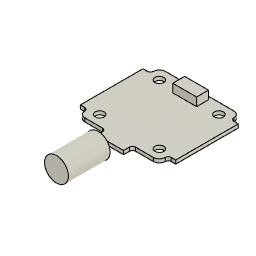
15A ESC v4 (Autodesk Fusion 360 design; units mm, degrees)
Autodesk Fusion 360 part; units mm, degrees
note: some values were not read from the file. Set by a fixed rule: which sketch regions a step uses.
sketch "Sketch1" plane through (0, 0, 0) normal (0, 0, 1) x (1, 0, 0)
  line L0 (-10, 10) -> (10, 10) construction
  line L1 (10, 10) -> (10, -10) construction
  line L2 (10, -10) -> (-10, -10) construction
  line L3 (-10, -10) -> (-10, 10) construction
  line L4 (-10, 10) -> (10, -10) construction
  line L5 (10, 10) -> (-10, -10) construction
  circle A0 centre (-10, 10) radius 1.5
  circle A1 centre (10, 10) radius 1.5
  circle A2 centre (10, -10) radius 1.5
  circle A3 centre (-10, -10) radius 1.5
  line L6 (-13.5, 13.5) -> (13.5, 13.5)
  line L7 (13.5, 13.5) -> (13.5, -13.5)
  line L8 (13.5, -13.5) -> (-13.5, -13.5)
  line L9 (-13.5, -13.5) -> (-13.5, 13.5)
  line L10 (-13.5, 13.5) -> (13.5, -13.5) construction
  line L11 (13.5, 13.5) -> (-13.5, -13.5) construction
  line L12 (-4.5, -16.5) -> (4.5, -16.5)
  line L13 (4.5, -16.5) -> (4.5, -13.5)
  line L14 (4.5, -13.5) -> (-4.5, -13.5)
  line L15 (-4.5, -13.5) -> (-4.5, -16.5)
  line L16 (-16, 10.5) -> (-13.5, 10.5)
  line L17 (-13.5, 10.5) -> (-13.5, -10.5)
  line L18 (-13.5, -10.5) -> (-16, -10.5)
  line L19 (-16, -10.5) -> (-16, 10.5)
  line L20 (0, 2.5) -> (0, 20)
  line L21 (13.5, 10.5) -> (13.5, -10.5)
  line L22 (13.5, -10.5) -> (16, -10.5)
  line L23 (16, -10.5) -> (16, 10.5)
  line L24 (16, 10.5) -> (13.5, 10.5)
  line L25 (-4, 12.5) -> (4, 12.5)
  line L26 (4, 12.5) -> (4, 8.5)
  line L27 (4, 8.5) -> (-4, 8.5)
  line L28 (-4, 8.5) -> (-4, 12.5)
  line L29 (-4, 12.5) -> (4, 8.5) construction
  line L30 (4, 12.5) -> (-4, 8.5) construction
  point P0 (0, 10.5)
  dimension "d1" = 20
  dimension "d2" = 20
  dimension "d3" = 3
  dimension "d4" = 27
  dimension "d5" = 27
  dimension "d6" = 9
  dimension "d7" = 3
  dimension "d8" = 2.5
  dimension "d9" = 21
  dimension "d12" = 8
  dimension "d13" = 4
  dimension "d14" = 1
  constraint horizontal L0
  constraint perpendicular L0 L1
  constraint parallel L0 L2
  constraint parallel L1 L3
  constraint coincident L4 origin
  constraint coincident L5 origin
  constraint coincident L0.start L3.end
  constraint coincident L0.end L1.start
  constraint coincident L1.end L2.start
  constraint coincident L2.end L3.start
  constraint equal A1 A3
  constraint equal A1 A2
  constraint equal A0 A2
  constraint horizontal L6
  constraint perpendicular L6 L7
  constraint parallel L6 L8
  constraint parallel L7 L9
  constraint coincident L10 origin
  constraint coincident L11 origin
  constraint horizontal L12
  constraint vertical L13
  constraint horizontal L14
  constraint vertical L15
  constraint midpoint L8 L14
  constraint horizontal L16
  constraint vertical L17
  constraint horizontal L18
  constraint vertical L19
  constraint midpoint L9 L17
  constraint symmetric L16.start L20 L23.end
  constraint symmetric L16.end L20 L21.start
  constraint symmetric L17.end L20 L21.end
  constraint symmetric L18.end L20 L22.end
  constraint horizontal L25
  constraint perpendicular L25 L26
  constraint parallel L25 L27
  constraint parallel L26 L28
  constraint coincident L29 P0
  constraint coincident L30 P0
  constraint coincident L20 P0
  measures "d1" distance of L1.end L2.end
  measures "d2" distance of L0.end L1.end
  measures "d3" diameter of A0
  measures "d4" distance of L7.end L8.end
  measures "d5" distance of L6.end L7.end
  measures "d6" distance of L12.start L12.end
  measures "d7" distance of L12.start L14.end
  measures "d8" distance of L16.start L16.end
  measures "d9" distance of L16.start L18.end
  measures "d12" distance of L26.end L27.end
  measures "d13" distance of L25.end L26.end
  measures "d14" distance of L6 L25
extrude "Extrude1" add sketch "Sketch1" along normal blind 1.2 makes body 1
extrude "Extrude2" add sketch "Sketch1" along normal blind 4 contours L20 L25 L27 L28 | L20 L25 L26 L27 bodies 1
fillet "Fillet1" radius 1 6 edges at (4.5, -13.5, 0.6) (-4.5, -13.5, 0.6) (-13.5, -10.5, 0.6) (-13.5, 10.5, 0.6) (13.5, 10.5, 0.6) (13.5, -10.5, 0.6) on bodies 1
fillet "Fillet2" radius 2 4 edges at (-13.5, -13.5, 0.6) (13.5, -13.5, 0.6) (13.5, 13.5, 0.6) (-13.5, 13.5, 0.6) on bodies 1
sketch "Sketch2" plane through (0, -16.5, 0) normal (0, -1, 0) x (1, 0, 0)
  line L0 (-4.5, 0) -> (4.5, 0)
  line L1 (4.5, 0) -> (4.5, 1.2)
  line L2 (4.5, 1.2) -> (-4.5, 1.2)
  line L3 (-4.5, 1.2) -> (-4.5, 0)
  circle A0 centre (0, 2.5) radius 4
  line L4 (0, 2.5) -> (0, 0) construction
  dimension "d23" = 8
  dimension "d24" = 2.5
  constraint coincident A0.centre L4.start
  constraint coincident L4.end origin
  constraint perpendicular L0 L4
  measures "d23" diameter of A0
  measures "d24" distance of L4.end A0.centre
extrude "Extrude3" add sketch "Sketch2" along normal blind 1 and the other way blind -15 separate body contours L0 L2 A0 | L0 A0 | L2 A0 makes body 2
move_body "Move1" bodies 2 to x (1, 0, 0) y (0, 1, 0) z (0, 0, 1) at (0, -3, 0)
